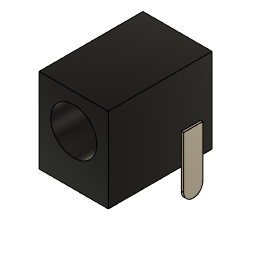
WLED_MiniDuo_CASE (Autodesk Fusion 360 archive; units mm, degrees)
design "DC Jack"
Autodesk Fusion 360 part; units mm, degrees
sketch "Sketch1" plane through (0, 0, 0) normal (0, 0, 1) x (1, 0, 0)
  line L0 (-4.5, 6.75) -> (4.5, 6.75)
  line L1 (4.5, 6.75) -> (4.5, -6.75)
  line L2 (4.5, -6.75) -> (-4.5, -6.75)
  line L3 (-4.5, -6.75) -> (-4.5, 6.75)
  line L4 (-4.5, 6.75) -> (4.5, -6.75) construction
  line L5 (4.5, 6.75) -> (-4.5, -6.75) construction
  dimension "d1" = 9
  dimension "d2" = 13.5
  constraint horizontal L0
  constraint perpendicular L0 L1
  constraint parallel L0 L2
  constraint parallel L1 L3
  constraint coincident L4 origin
  constraint coincident L5 origin
  measures "d1" distance of L1.end L2.end
  measures "d2" distance of L0.end L1.end
extrude "Extrude1" add sketch "Sketch1" along normal blind 11 makes body 1
sketch "Sketch2" plane through (0, -6.75, 0) normal (0, -1, 0) x (1, 0, 0)
  line L0 (-4.5, 0) -> (4.5, 0)
  line L1 (4.5, 0) -> (4.5, 11)
  line L2 (4.5, 11) -> (-4.5, 11)
  line L3 (-4.5, 11) -> (-4.5, 0)
  circle A0 centre (0, 6.5) radius 3
  dimension "d5" = 6.5
  dimension "d6" = 6
  constraint vertical origin A0.centre
  measures "d5" distance of origin A0.centre
  measures "d6" diameter of A0
extrude "Extrude2" cut sketch "Sketch2" against normal blind 11 contours A0 bodies 1
sketch "Sketch3" plane through (0, 6.75, 0) normal (0, 1, 0) x (-1, 0, 0)
  line L0 (-4.5, 0) -> (4.5, 0) construction
  line L1 (4.5, 0) -> (4.5, 11) construction
  line L2 (4.5, 11) -> (-4.5, 11) construction
  line L3 (-4.5, 11) -> (-4.5, 0) construction
  circle A0 centre (0, 6.5) radius 3 construction
  line L4 (-1.25, 6.5) -> (-1.25, -2.75)
  arc A1 (-1.25, -2.75) -> (1.25, -2.75) centre (0, -2.75) ccw
  line L5 (1.25, -2.75) -> (1.25, 6.5)
  arc A2 (1.25, 6.5) -> (-1.25, 6.5) centre (0, 6.5) ccw
  dimension "d9" = 2.5
  dimension "d10" = 2.75
  constraint tangent L4 A1
  constraint tangent A1 L5
  constraint parallel L4 L5
  constraint tangent L5 A2
  constraint tangent L4 A2
  constraint vertical A1.centre A0.centre
  constraint coincident A0.centre A2.centre
  measures "d9" distance of L4 L5
  measures "d10" distance of L0 A1.centre
extrude "Extrude3" add sketch "Sketch3" along normal blind 0.3 separate body makes body 2
sketch "Sketch4" plane through (4.5, 0, 0) normal (1, 0, 0) x (0, 1, 0)
  line L0 (-6.75, 0) -> (6.75, 0) construction
  line L1 (6.75, 0) -> (6.75, 11) construction
  line L2 (6.75, 11) -> (-6.75, 11) construction
  line L3 (-6.75, 11) -> (-6.75, 0) construction
  line L4 (2.75, 4) -> (5.25, 4)
  line L5 (5.25, 4) -> (5.25, -2.75)
  arc A0 (2.75, -2.75) -> (5.25, -2.75) centre (4, -2.75) ccw
  line L6 (2.75, -2.75) -> (2.75, 4)
  dimension "d13" = 2.5
  dimension "d14" = 2.75
  dimension "d15" = 10.75
  dimension "d16" = 4
  constraint horizontal L4
  constraint tangent L5 A0
  constraint tangent A0 L6
  constraint perpendicular L4 L5
  constraint perpendicular L4 L6
  measures "d13" distance of L4.start L4.end
  measures "d14" distance of L0 A0.centre
  measures "d15" distance of L3 A0.centre
  measures "d16" distance of L0 L4
extrude "Extrude4" add sketch "Sketch4" along normal blind 0.3 separate body makes body 3
ref_plane "WorkPlane1" through (0, 0.75, 1.875) normal (0, -1, 0) x (1, 0, 0)
sketch "Sketch5" plane through (0, 0.75, 1.875) normal (0, -1, 0) x (1, 0, 0)
  arc A0 (1.25, 4.625) -> (-1.25, 4.625) centre (0, 4.625) ccw
  line L0 (-1.25, 4.625) -> (-1.25, -4.625)
  arc A1 (-1.25, -4.625) -> (1.25, -4.625) centre (0, -4.625) ccw
  line L1 (1.25, -4.625) -> (1.25, 4.625)
  line L2 (-4.5, -1.875) -> (4.5, -1.875)
extrude "Extrude5" add sketch "Sketch5" along normal blind 0.3 separate body contours L0 A1 L1 L2 makes body 4
equation "d10 = 4 mm - ( 2.5 / 2 ) * 1 mm"
equation "d14 = 4 mm - ( 2.5 / 2 ) * 1 mm"
named bodies: "Body", "Center Lead", "Side Lead", "Bottom Lead"
